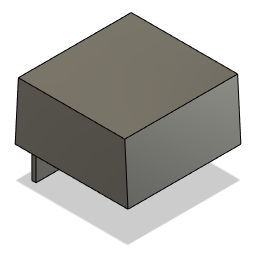
Raspi Pisugar and LED Driver (Autodesk Fusion 360 archive; units mm, degrees)
design "BuckPuck LED Driver"
Autodesk Fusion 360 part; units mm, degrees
sketch "Front View" plane through (0, 0, 0) normal (0, 0, 1) x (1, 0, 0)
  line L0 (0, 0) -> (21, 0)
  line L1 (0.6, 11) -> (20.4, 11)
  line L2 (0.6, 11) -> (0, 0)
  line L3 (20.4, 11) -> (21, 0)
  dimension "d1" = 21
  dimension "d2" = 19.8
  dimension "d3" = 11
  constraint coincident L0.start L2.end
  constraint horizontal L0
  measures "d1" distance of L0.start L0.end
  measures "d2" distance of L1.start L1.end
  measures "d3" distance of L0 L1
extrude "Extrude1" add sketch "Front View" against normal blind 21
sketch "Pin Sketches" plane through (0, 0, 0) normal (0, -1, 0) x (1, 0, 0)
  line L0 (21, 0) -> (0, 0)
  line L1 (0, 0) -> (0, -21)
  line L2 (0, -21) -> (21, -21)
  line L3 (21, -21) -> (21, 0)
  line L4 (1.62, -18.88) -> (2.38, -18.88)
  line L5 (2.38, -18.88) -> (2.38, -18.12)
  line L6 (2.38, -18.12) -> (1.62, -18.12)
  line L7 (1.62, -18.12) -> (1.62, -18.88)
  line L8 (1.62, -18.88) -> (2.38, -18.88)
  line L9 (2.38, -18.88) -> (2.38, -1.5)
  line L10 (2.38, -1.5) -> (1.62, -1.5)
  line L11 (1.62, -1.5) -> (1.62, -18.88)
  dimension "d6" = 0.76
  dimension "d7" = 0.76
  dimension "d8" = 1.62
  dimension "d9" = 2.12
  constraint horizontal L4
  constraint vertical L5
  constraint horizontal L6
  constraint vertical L7
  constraint horizontal L8
  constraint vertical L9
  constraint horizontal L10
  constraint vertical L11
  measures "d6" distance of L4.start L6.end
  measures "d7" distance of L5.end L6.end
  measures "d8" distance of L1 L7
  measures "d9" distance of L2 L4
extrude "Extrude2" add sketch "Pin Sketches" along normal blind 5.8 contours L4 L5 L6 L7 L8 L9 L11 | L6 L9 L10 L11
